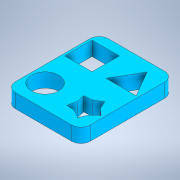
# Autodesk Inventor part: PassengerBaseGBR
Saved by Autodesk Inventor 2020.1 (Build 241239000, 239)
## iProperties
Created: 2020-03-09
Part Number: PassengerBaseGBR
Material: Generic
Document SubType Name: Modeling
Designer: super
Density: 1 g/cm^3
Appearance: Default
Author: super
Autodesk Inventor part; units mm, degrees
ref_plane "YZ Plane" through (0, 0, 0) normal (1, 0, 0) x (0, 1, 0)
ref_plane "XZ Plane" through (0, 0, 0) normal (0, 1, 0) x (-1, 0, 0)
ref_plane "XY Plane" through (0, 0, 0) normal (0, 0, 1) x (1, 0, 0)
sketch "Sketch1" plane through (0, 0, 0) normal (0, 1, 0) x (-1, 0, 0)
  line L0 (0, 0) -> (-40.386, 0)
  line L1 (-40.386, 0) -> (-40.386, -50.165)
  line L2 (-40.386, -50.165) -> (0, -50.165)
  circle A0 centre (-8.636, -12.446) radius 7.366
  line L3 (-1.27, -45.085) -> (-1.27, -30.353)
  line L4 (-1.27, -30.353) -> (-16.002, -30.353)
  line L5 (-16.002, -30.353) -> (-16.002, -45.085)
  line L6 (-16.002, -45.085) -> (-1.27, -45.085)
  line L7 (-31.0134, -45.085) -> (-22.9108, -31.0509)
  line L8 (-22.9108, -31.0509) -> (-39.116, -31.0509)
  line L9 (-39.116, -31.0509) -> (-31.0134, -45.085)
  line L10 (-40.386, 0) -> (-40.386, -12.3952)
  line L11 (-38.8493, -12.3952) -> (-35.3989, -15.4707)
  line L12 (-33.5401, -19.7026) -> (-35.3989, -15.4707)
  line L13 (-24.9497, -7.879) -> (-25.9334, -12.3952)
  line L14 (-24.9497, -16.9114) -> (-25.9334, -12.3952)
  line L15 (-24.9497, -16.9114) -> (-29.2449, -17.2623)
  line L16 (-33.5401, -19.7026) -> (-29.2449, -17.2623)
  line L17 (-33.5401, -5.0878) -> (-29.2449, -7.5281)
  line L18 (-24.9497, -7.879) -> (-29.2449, -7.5281)
  line L19 (-38.8493, -12.3952) -> (-35.3989, -9.3197)
  line L20 (-33.5401, -5.0878) -> (-35.3989, -9.3197)
  line L21 (0, -50.165) -> (0, 0)
  point P0 (-31.1658, -12.3952)
  dimension "d0" = 40.386
  dimension "d1" = 50.165
  dimension "d4" = 14.732
  dimension "d7" = 14.732
  dimension "d8" = 14.732
  dimension "d15" = 12.3952
  constraints: 44 end point, 2 perpendicular, 1 centre point, 1 horizontal, 1 parallel, 1 point on line, 1 vertical, 6 other
  measures "d0" distance of L2.end L1.end
  measures "d1" distance of L1.end L0.end
  measures "d4" diameter of A0
  measures "d7" distance of L3.start L3.end
  measures "d8" distance of L3.end L4.end
  measures "d15" distance of L0.end L10.end
extrude "Extrusion1" add sketch "Sketch1" along normal blind 7.62
fillet "Fillet1" radius 5.08 4 edges at (40.386, 3.81, 0) (40.386, 3.81, -50.165) (0, 3.81, -50.165) (0, 3.81, 0)
shell "Shell1" thickness 0.254 removed faces 1 at (23.3087, 0, -40.407)
body "Solid1"
